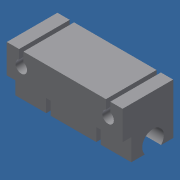
# Autodesk Inventor part: GantryHolder
Saved by Autodesk Inventor 2018 (Build 220112000, 112)
## iProperties
Created: 2022-08-28
Part Number: GantryHolder
Material: Generic
Document SubType Name: Modeling
Designer: Nathann
Density: 1 g/cm^3
Appearance: Default
Author: Nathann
Autodesk Inventor part; units mm, degrees
ref_plane "YZ Plane" through (0, 0, 0) normal (1, 0, 0) x (0, 1, 0)
ref_plane "XZ Plane" through (0, 0, 0) normal (0, 1, 0) x (-1, 0, 0)
ref_plane "XY Plane" through (0, 0, 0) normal (0, 0, 1) x (1, 0, 0)
sketch "Sketch1" plane through (0, 0, 0) normal (0, 1, 0) x (-1, 0, 0)
  arc A0 (8.5, 13.7081) -> (11.5, 13.7081) centre (10, 10) ccw
  line L0 (8.5, 20) -> (8.5, 13.7081)
  line L1 (11.5, 20) -> (11.5, 13.7081)
  line L2 (10, 20) -> (10, 18.7339)
  line L3 (20, 20) -> (10, 20)
  line L4 (8.5, 20) -> (0, 20)
  line L5 (0, 20) -> (0, 0)
  line L6 (0, 0) -> (20, 0)
  line L7 (20, 0) -> (20, 20)
  arc A1 (68.5, 13.7081) -> (71.5, 13.7081) centre (70, 10) ccw
  line L8 (68.5, 20) -> (68.5, 13.7081)
  line L9 (71.5, 20) -> (71.5, 13.7081)
  line L10 (70, 20) -> (70, 18.3732)
  line L11 (80, 20) -> (70, 20)
  line L12 (68.5, 20) -> (60.9559, 20)
  line L13 (60.9559, 20) -> (60.9559, 0)
  line L14 (60.9559, 0) -> (80, 0)
  line L15 (80, 0) -> (80, 20)
  line L16 (60.9559, 0) -> (20, 0)
  line L17 (20, 0) -> (20, 20)
  line L18 (20, 20) -> (60.9559, 20)
  line L19 (60.9559, 20) -> (60.9559, 0)
  dimension "d2" = 8
  dimension "d7" = 1.5
  dimension "d8" = 1.5
  dimension "d16" = 10
  dimension "d17" = 8
  dimension "d18" = 1.5
  dimension "d19" = 1.5
  dimension "d20" = 10
  dimension "d22" = 80
  dimension "d23" = 10
  dimension "d24" = 0
  dimension "d25" = 60
  dimension "d26" = 20
  dimension "d27" = 20
  dimension "d28" = 20
  dimension "d29" = 20
  dimension "d30" = 10
  dimension "d31" = 10
  dimension "d32" = 20
  constraints: 40 end point, 6 vertical, 5 perpendicular, 4 parallel, 4 point on circle, 3 point on line, 2 centre point, 1 horizontal
  measures "d2" diameter of A0
  measures "d7" distance between parallel lines of L0 L2
  measures "d8" distance between parallel lines of L1 L2
  measures "d16" horizontal distance of L5.end A0.centre
  measures "d17" diameter of A1
  measures "d18" distance between parallel lines of L8 L10
  measures "d19" distance between parallel lines of L9 L10
  measures "d20" vertical distance of L13.end A1.centre
  measures "d22" distance between parallel lines of L5 L15
  measures "d23" distance from line of L15 A1.centre
  measures "d24" distance between parallel lines of L6 L14
  measures "d25" distance of A0.centre A1.centre
  measures "d26" distance of L14.end L11.start
  measures "d27" distance of L12.end L13.end
  measures "d28" distance of L6.end L3.start
  measures "d29" distance of L4.end L5.end
  measures "d30" distance between parallel lines of L15 L10
  measures "d31" distance between parallel lines of L7 L2
  measures "d32" distance between parallel lines of L16 L18
extrude "Extrusion1" add sketch "Sketch1" along normal blind 36
sketch "Sketch5" plane through (-80, 0, 0) normal (-1, 0, 0) x (0, 0, 1)
  line L0 (20, 0) -> (20, 36) projected
  line L1 (20, 36) -> (-15, 36)
  line L2 (-15, 6) -> (20, 6)
  line L3 (20, 6) -> (20, 36)
  line L4 (-15, 36) -> (-15, 26.6522)
  line L5 (-15, 15.4718) -> (-15, 6)
  line L6 (0, 0) -> (0, 36) projected
  line L7 (0, 0) -> (0, 36) projected
  line L8 (0, 6) -> (0, 36)
  arc A0 (-15, 15.4718) -> (-15, 26.6522) centre (-10, 21.062) ccw
  dimension "d40" = 30
  dimension "d41" = 35
  dimension "d45" = 20
  dimension "d85" = 15
  dimension "d86" = 5
  dimension "d87" = 15
  constraints: 12 end point, 3 parallel, 2 perpendicular, 2 point on circle, 2 point on line, 1 centre point, 1 horizontal, 1 vertical
  measures "d40" distance of L1.end L2.start
  measures "d41" distance of L0.end L1.end
  measures "d45" distance between parallel lines of L0 L6
  measures "d85" diameter of A0
  measures "d86" distance from line of L4 A0.centre
  measures "d87" distance between parallel lines of L6 L5
extrude "Extrusion5" add sketch "Sketch5" against normal blind 80 contours L2 L5 A0 L4 L1 L6
sketch "Sketch13" plane through (0, 36, 0) normal (0, 1, 0) x (1, 0, 0)
  line L0 (-80, -20) -> (-80, 15) projected
  line L1 (-80, -20) -> (-71.5, -20) projected
  line L2 (-71.5, -20) -> (-71.5, -13.7081) projected
  arc A0 (-68.5, -13.7081) -> (-71.5, -13.7081) centre (-70, -10) ccw projected
  line L3 (-68.5, -13.7081) -> (-68.5, -20) projected
  line L4 (-68.5, -20) -> (-11.5, -20) projected
  line L5 (-11.5, -20) -> (-11.5, -13.7081) projected
  arc A1 (-8.5, -13.7081) -> (-11.5, -13.7081) centre (-10, -10) ccw projected
  line L6 (-8.5, -13.7081) -> (-8.5, -20) projected
  line L7 (-8.5, -20) -> (0, -20) projected
  line L8 (0, -20) -> (0, 15) projected
  line L9 (-80, 15) -> (0, 15) projected
  point P0 (0, 0)
extrude "Extrusion11" cut sketch "Sketch13" against normal blind 1
equation "\"d2\" = RodDiameter"
equation "\"d17\" = d2"
equation "\"RodDiameter\" = 8"
equation "\"VerticalBearingOD\" = 16"
equation "\"PrintingClearance\" = 0.2"
equation "\"d21\" = 8"
body "Solid1"
